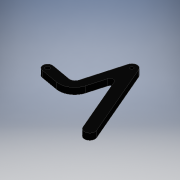
# Autodesk Inventor part: Leg3
Saved by Autodesk Inventor 2016 (Build 200138000, 138)
## iProperties
Created: 2015-12-10
Part Number: Leg3
Material: Generic
Document SubType Name: Modeling
Designer: lk8187
Density: 1 g/cm^3
Appearance: Smooth - Black(1)
Author: lk8187
Autodesk Inventor part; units mm, degrees
ref_plane "YZ Plane" through (0, 0, 0) normal (1, 0, 0) x (0, 1, 0)
ref_plane "XZ Plane" through (0, 0, 0) normal (0, 1, 0) x (-1, 0, 0)
ref_plane "XY Plane" through (0, 0, 0) normal (0, 0, 1) x (1, 0, 0)
sketch "Sketch1" plane through (0, 0, 0) normal (0, 0, 1) x (1, 0, 0)
  circle A0 centre (0, 0) radius 2
  arc A1 (0.7814, 4.4316) -> (-0.7814, -4.4316) centre (0, 0) ccw
  arc A2 (44.5957, 41.9696) -> (35.1896, 41.3639) centre (40, 40) ccw
  line L0 (44.5957, 41.9696) -> (74.5957, -28.0304)
  arc A3 (65.4043, -31.9696) -> (74.5957, -28.0304) centre (70, -30) ccw
  circle A4 centre (40, 40) radius 1.5
  line L1 (0, 0) -> (46.8621, 0) construction
  line L2 (65.4043, -31.9696) -> (43.0454, 20.2011)
  line L3 (0.7814, 4.4316) -> (19.1318, 1.196)
  arc A5 (19.1318, 1.196) -> (24.8104, 4.7561) centre (20, 6.12) ccw
  line L4 (24.8104, 4.7561) -> (35.1896, 41.3639)
  line L5 (-0.7814, -4.4316) -> (15.6896, -7.3359)
  arc A6 (15.6896, -7.3359) -> (32.7255, 3.3446) centre (18.2943, 7.4362) ccw
  line L6 (32.7255, 3.3446) -> (37.4017, 19.8377)
  arc A7 (43.0454, 20.2011) -> (37.4017, 19.8377) centre (40.288, 19.0194) ccw
  dimension "d0" = 4
  dimension "d1" = 3
  dimension "d2" = 4.5
  dimension "d5" = 40
  dimension "d6" = 5
  dimension "d8" = 10
  dimension "d9" = 40
  dimension "d10" = 30
  dimension "d11" = 70
  dimension "d12" = 10
  dimension "d13" = 20
  dimension "d14" = 8
  dimension "d15" = 5
  dimension "d16" = 15
  dimension "d17" = 3
  constraints: 14 end point, 12 point on circle, 12 tangent, 8 centre point, 3 coincident, 3 parallel, 1 horizontal
  measures "d0" diameter of A0
  measures "d1" diameter of A4
  measures "d2" radius of A1
  measures "d5" distance from line of L1 A2.centre
  measures "d6" radius of A2
  measures "d8" distance between parallel lines of L0 L2
  measures "d9" horizontal distance of A2.centre point (0, 0)
  measures "d10" distance from line of A3.centre L1
  measures "d11" horizontal distance of A3.centre point (0, 0)
  measures "d12" angle of L3 L1
  measures "d13" horizontal distance of point (0, 0) A5.centre
  measures "d14" distance between parallel lines of L4 L6
  measures "d15" radius of A5
  measures "d16" radius of A6
  measures "d17" radius of A7
extrude "Extrusion1" add sketch "Sketch1" along normal blind 6
body "Solid1"
